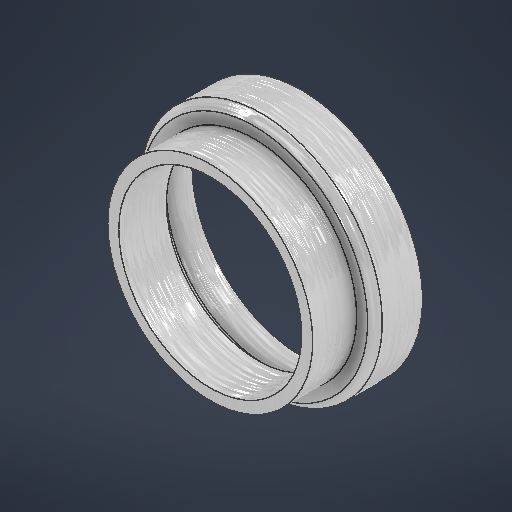
# Autodesk Inventor part: EXTRUSSOR-COUPLING
Saved by Autodesk Inventor 2025.3 (Build 293356030, 356C)
## iProperties
Created: 2025-09-01
Part Number: EXTRUSSOR-COUPLING
Material: Generic
Document SubType Name: Modeling
Designer: lstk1ng
Density: 1 g/cm^3
Appearance: Polished Brushed
Author: lstk1ng
Autodesk Inventor part; units mm, degrees
ref_plane "YZ Plane" through (0, 0, 0) normal (1, 0, 0) x (0, 1, 0)
ref_plane "XZ Plane" through (0, 0, 0) normal (0, 1, 0) x (-1, 0, 0)
ref_plane "XY Plane" through (0, 0, 0) normal (0, 0, 1) x (1, 0, 0)
sketch "Sketch1" plane through (0, 0, 0) normal (0, 1, 0) x (-1, 0, 0)
  line L0 (0, 26.3121) -> (0, -23.4342)
  line L1 (30, -13.4342) -> (30, -3.4342)
  line L2 (25, -1.4342) -> (25, 11.5658)
  line L3 (30, -3.4342) -> (27, -3.4342)
  line L4 (28, 11.5658) -> (28, -0.4342)
  line L5 (28, -0.4342) -> (31, -0.4342)
  line L6 (33, -2.4342) -> (33, -13.4342)
  line L7 (28, 11.5658) -> (25, 11.5658)
  line L8 (27, -3.4342) -> (25, -1.4342)
  line L9 (33, -2.4342) -> (31, -0.4342)
  line L10 (30, -3.4342) -> (30, -13.4342)
  line L11 (30, -13.4342) -> (33, -13.4342)
  point P0 (0, 0)
  point P1 (25, -3.4342)
  point P2 (33, -0.4342)
  dimension "d1" = 60
  dimension "d2" = 15
  dimension "d3" = 50
  dimension "d4" = 2
  dimension "d5" = 2
  dimension "d6" = 2
  dimension "d7" = 2
  constraints: 24 end point, 4 point on line, 4 vertical, 2 horizontal, 1 collinear, 1 perpendicular
  measures "d1" diameter of L1.start L0
  measures "d2" distance of point (25, -3.434) L2.end
  measures "d3" diameter of L2 L0
  measures "d4" distance of L3.end point (25, -3.434)
  measures "d5" distance of L2.start point (25, -3.434)
  measures "d6" distance of L6.start point (33, -0.434)
  measures "d7" distance of L5.end point (33, -0.434)
revolve "Revolution1" add sketch "Sketch1" angle 360 about axis through (0, 0, 26.3121) along (0, 0, -1)
equation "\"d5\" = d4"
equation "\"d7\" = d6"
body "Solid1"
